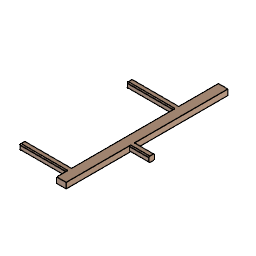
furca (Autodesk Fusion 360 design; units mm, degrees)
part number: 2026-06-02-07-13-39-938
Autodesk Fusion 360 part; units mm, degrees
note: some values were not read from the file. Set by a fixed rule: which sketch regions a step uses.
sketch "Sketch1" plane through (0, 0, 0) normal (0, 0, 1) x (1, 0, 0)
  line L0 (-1.25, 17.5) -> (1.25, 17.5)
  line L1 (1.25, 17.5) -> (1.25, -17.5)
  line L2 (1.25, -17.5) -> (-1.25, -17.5)
  line L3 (-1.25, -17.5) -> (-1.25, 17.5)
  line L4 (-1.25, 17.5) -> (1.25, -17.5) construction
  line L5 (1.25, 17.5) -> (-1.25, -17.5) construction
  line L6 (0, 0) -> (0, -14.0845) construction
  line L7 (-1.25, -14.8345) -> (-13.75, -14.8345)
  line L8 (-13.75, -14.8345) -> (-13.75, -13.3345)
  line L9 (-13.75, -13.3345) -> (-1.25, -13.3345)
  line L10 (1.25, -0.775) -> (6.25, -0.775)
  line L11 (6.25, -0.775) -> (6.25, 0.725)
  line L12 (6.25, 0.725) -> (1.25, 0.725)
  line L13 (0, -14.0845) -> (-12.5, -14.0845) construction
  line L14 (0, 0) -> (-10.5, 0) construction
  line L15 (-13.75, 13.3345) -> (-1.25, 13.3345)
  line L16 (-1.25, 14.8345) -> (-13.75, 14.8345)
  line L17 (-13.75, 13.3345) -> (-13.75, 14.8345)
  line L18 (-1.25, 17.5) -> (-1.25, 25)
  line L19 (1.25, 17.5) -> (1.25, 25)
  line L20 (1.25, 25) -> (-1.25, 25)
  dimension "d1" = 35
  dimension "d2" = 14.0845
  dimension "d3" = 0.75
  dimension "d4" = 1.5
  dimension "d5" = 12.5
  dimension "d6" = 1.5
  dimension "d7" = 0.775
  dimension "d8" = 5
  dimension "d9" = 2.5
  dimension "d10" = 12.5
  dimension "d19" = 7.5
  dimension "d20" = 7.5
  constraint horizontal L0
  constraint perpendicular L0 L1
  constraint parallel L0 L2
  constraint parallel L1 L3
  constraint coincident L4 L6.start
  constraint coincident L5 L6.start
  constraint coincident L6.start L14.start
  constraint parallel L3 L6
  constraint coincident L3 L7.start
  constraint perpendicular L3 L7
  constraint perpendicular L7 L8
  constraint coincident L3 L9.end
  constraint perpendicular L3 L9
  constraint coincident L1 L10.start
  constraint perpendicular L1 L10
  constraint perpendicular L10 L11
  constraint coincident L1 L12.end
  constraint perpendicular L1 L12
  constraint perpendicular L6 L13
  constraint perpendicular L6 L14
  constraint symmetric L7.start L14 L16.start
  constraint symmetric L7.end L14 L16.end
  constraint symmetric L8.end L14 L15.start
  constraint symmetric L9.end L14 L15.end
  constraint perpendicular L0 L18
  constraint perpendicular L0 L19
  measures "d1" distance of L0.end L1.end
  measures "d2" distance of L6.start L6.end
  measures "d3" distance of L6.end L7
  measures "d4" distance of L7.end L8.end
  measures "d5" distance of L7.start L7.end
  measures "d6" distance of L10.end L11.end
  measures "d7" distance of L6.start L10
  measures "d8" distance of L1 L11
  measures "d9" distance of L1.end L2.end
  measures "d10" distance of L6.end L13.end
  measures "d19" distance of L0.start L18.end
  measures "d20" distance of L0.end L19.end
extrude "Extrude1" add sketch "Sketch1" along normal blind 1.5
fillet "Fillet1" radius 0.25 4 edges at (3.75, -0.775, 1.5) (3.75, -0.775, 0) (3.75, 0.725, 0) (3.75, 0.725, 1.5)
fillet "Fillet2" radius 0.25 4 edges at (-7.5, -14.8345, 1.5) (-7.5, -13.3345, 1.5) (-7.5, -13.3345, 0) (-7.5, -14.8345, 0)
fillet "Fillet3" radius 0.25 4 edges at (-7.5, 14.8345, 1.5) (-7.5, 13.3345, 1.5) (-7.5, 14.8345, 0) (-7.5, 13.3345, 0)
fillet "Fillet4" radius 0.25 16 edges at (-13.75, -14.8345, 0.75) (-13.75, -14.7613, 0.0732) (-13.75, -14.0845, 0) (-13.75, -13.4077, 0.0732) (-13.75, -13.3345, 0.75) (-13.75, -13.4077, 1.4268) (-13.75, -14.0845, 1.5) (-13.75, -14.7613, 1.4268) (-13.75, 13.3345, 0.75) (-13.75, 13.4077, 0.0732) (-13.75, 14.0845, 0) (-13.75, 14.7613, 0.0732) (-13.75, 14.8345, 0.75) (-13.75, 14.7613, 1.4268) (-13.75, 14.0845, 1.5) (-13.75, 13.4077, 1.4268)
equation "d2 = ( 28.169 / 2 ) * 1 mm"
equation "d3 = ( 1.5 / 2 ) * 1 mm"
equation "d7 = ( 1.55 / 2 ) * 1 mm"
named bodies: "furca"
